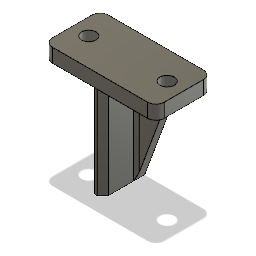
belt_tension_marker v3 (Autodesk Fusion 360 design; units mm, degrees)
Autodesk Fusion 360 part; units mm, degrees
sketch "Sketch2" plane through (0, 0, 0) normal (0, 1, 0) x (1, 0, 0)
  line L0 (20, 10) -> (-20, 10)
  line L1 (-20, 10) -> (-20, -10)
  line L2 (-20, -10) -> (20, -10)
  line L3 (20, -10) -> (20, 10)
  line L4 (20, 10) -> (-20, -10) construction
  line L5 (-20, 10) -> (20, -10) construction
  line L6 (-7, -10) -> (-7, 10)
  line L7 (-4, -10) -> (-4, 10)
  line L8 (-7, 7) -> (10, 7)
  line L9 (10, 7) -> (10, 10)
  line L10 (10, 10) -> (-7, 10)
  line L11 (-20, 0) -> (20, 0) construction
  circle A0 centre (-14, 0) radius 2.55
  circle A1 centre (14, 0) radius 2.55
  line L12 (-4, -5) -> (-7, -5)
  dimension "d1" = 20
  dimension "d2" = 3
  dimension "d3" = 3
  dimension "d10" = 40
  dimension "d11" = 5.1
  dimension "d12" = 5.1
  dimension "d13" = 6
  dimension "d14" = 6
  dimension "d17" = 17
  dimension "d19" = 4
  dimension "d23" = 5
  constraint horizontal L0
  constraint perpendicular L0 L1
  constraint parallel L0 L2
  constraint parallel L1 L3
  constraint coincident L4 origin
  constraint coincident L5 origin
  constraint coincident L2 L6.start
  constraint coincident L0 L6.end
  constraint perpendicular L0 L6
  constraint coincident L2 L7.start
  constraint coincident L0 L7.end
  constraint perpendicular L0 L7
  constraint coincident L6 L8.start
  constraint perpendicular L6 L8
  constraint perpendicular L8 L9
  constraint coincident L6 L10.end
  constraint perpendicular L6 L10
  constraint midpoint L1 L11.start
  constraint midpoint L3 L11.end
  constraint coincident L11 A0.centre
  constraint coincident L11 A1.centre
  constraint coincident L7 L12.start
  constraint coincident L6 L12.end
  constraint perpendicular L6 L12
  constraint collinear L0 L10
  measures "d1" distance of L0.start L2.end
  measures "d2" distance of L6 L7
  measures "d3" distance of L8.end L9.end
  measures "d10" distance of L1 L3
  measures "d11" diameter of A0
  measures "d12" diameter of A1
  measures "d13" distance of L1 A0.centre
  measures "d14" distance of L3 A1.centre
  measures "d17" distance of L9.end L6.end
  measures "d19" distance of origin L7
  measures "d23" distance of origin L12
extrude "Extrude1" add sketch "Sketch2" against normal blind 5 contours L0 L2 L3 L7 L8 L9 | L0 L7 L8 L9 L10 | L0 L6 L7 L8 L10 | L2 L6 L7 L12 | L0 L1 L2 L6 | L6 L7 L8 L12 | A0 | A1
extrude "Extrude2" add sketch "Sketch2" against normal blind 43 contours L0 L7 L8 L9 L10 | L0 L6 L7 L8 L10 | L6 L7 L8 L12
sketch "Sketch3" plane through (0, 0, -7) normal (0, 0, 1) x (1, 0, 0)
  line L0 (-4, -5) -> (-4, -43)
  line L1 (-4, -43) -> (10, -43)
  line L2 (10, -43) -> (10, -5)
  line L3 (10, -5) -> (-4, -43)
  line L4 (10, -5) -> (-4, -5)
  line L5 (20, -5) -> (-20, -5)
  constraint coincident L2 L3.start
  constraint coincident L0.end L1.start
  constraint coincident L2.end L5
extrude "Extrude3" cut sketch "Sketch3" against normal through all contours L1 L2 L3
extrude "Extrude4" cut sketch "Sketch2" against normal through all contours A0 | A1
chamfer "Chamfer1" [suppressed]
fillet "Fillet1" radius 3 4 edges at (-20, -2.5, 10) (20, -2.5, 10) (20, -2.5, -10) (-20, -2.5, -10)
chamfer "Chamfer2" distance 1 angle 45 2 edges at (-7, -24, -10) (-4, -24, -7)
chamfer "Chamfer3" distance 2 angle 45 1 edges at (-4, -24, 5)
sketch "Sketch1" plane through (0, 0, 0) normal (0, 0, 1) x (1, 0, 0)
equation "d3 = d2"
equation "d12 = d11"
equation "d14 = d13"
